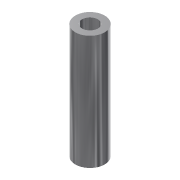
# Autodesk Inventor part: PP-01
Saved by Autodesk Inventor 2022 (Build 260148000, 148)
## iProperties
Created: 2008-09-23
Part Number: PP-01
Document SubType Name: Modeling
Designer: Mark Flayler
Mass: 0.0132542 g
Surface Area: 0.169966 cm^2
Volume: 0.00168628 cm^3
Density: 7.86 g/cm^3
Material: Steel, Mild
Description: LEAD GUIDE
Appearance: Aluminum - Polished
Author: Mark Flayler
Autodesk Inventor part; units mm, degrees
ref_plane "YZ Plane" through (0, 0, 0) normal (1, 0, 0) x (0, 1, 0)
ref_plane "XZ Plane" through (0, 0, 0) normal (0, 1, 0) x (-1, 0, 0)
ref_plane "XY Plane" through (0, 0, 0) normal (0, 0, 1) x (1, 0, 0)
sketch "Sketch1" plane through (0, 0, 0) normal (0, 0, 1) x (1, 0, 0)
  circle A0 centre (0, 0) radius 0.46
  circle A1 centre (0, 0) radius 0.25
  dimension "d0" = 0.92
  dimension "d2" = 0.5
  constraints: 2 centre point, 2 coincident
  measures "d0" diameter of A0
  measures "d2" diameter of A1
extrude "Extrusion1" add sketch "Sketch1" along normal blind 3.6
equation "\"User1\" = 1"
body "Solid1"
